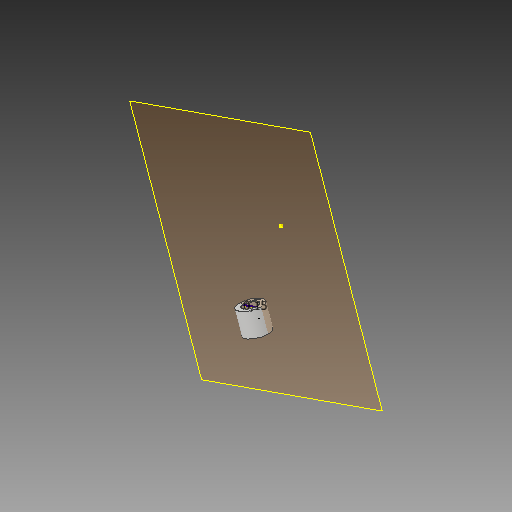
# Autodesk Inventor part: motor_handler
Saved by Autodesk Inventor 2019 (Build 230136000, 136)
## iProperties
Created: 2019-01-23
Part Number: motor_handler
Material: Generic
Document SubType Name: Modeling
Designer: jmc
Density: 1 g/cm^3
Appearance: Default
Author: jmc
Autodesk Inventor part; units mm, degrees
ref_plane "YZ Plane" through (0, 0, 0) normal (1, 0, 0) x (0, 1, 0)
ref_plane "XZ Plane" through (0, 0, 0) normal (0, 1, 0) x (-1, 0, 0)
ref_plane "XY Plane" through (0, 0, 0) normal (0, 0, 1) x (1, 0, 0)
ref_plane "Work Plane2" through (-89.4914, 16.4002, -46.0725) normal (0, 0, 1) x (0.3299211, -0.9440085, 0)
sketch "Sketch3" plane through (-89.4914, 16.4002, -46.0725) normal (0, 0, 1) x (0.3299211, -0.9440085, 0)
  line L0 (142.5, 12.3) -> (142.5, -12.3) projected
  line L1 (142.35, 11.9681) -> (142.35, -12.4873)
  point P0 (45.0071, 79.0699)
  dimension "d3" = 0.15
  constraints: 2 end point, 1 vertical
  measures "d3" distance between parallel lines of L1 L0
sketch "Sketch2" plane through (-89.4914, 16.4002, -46.0725) normal (0, 0, 1) x (0.3299211, -0.9440085, 0)
  line L0 (144.2, -14) -> (171.4, -14)
  line L1 (142.5, -12.3) -> (142.5, 11.0344) projected
  line L2 (130, 22) -> (130, -22) projected
  line L3 (144.2, 16.15) -> (171.4, 16.15)
  line L4 (171.4, 16.15) -> (171.4, 14.15)
  line L5 (144.2, 14.15) -> (171.4, 14.15)
  line L6 (156.1685, 0) -> (84.745, 0) construction
  line L7 (144.2, 14.15) -> (142.35, 14.15)
  line L8 (142.35, 16.15) -> (144.2, 16.15)
  line L9 (142.35, 11.9681) -> (142.35, -12.4873) projected
  line L10 (142.5, 14.15) -> (142.35, 14.15)
  line L11 (142.35, 14.15) -> (142.35, 16.15)
  line L12 (142.35, 16.15) -> (142.5, 16.15)
  point P0 (45.0071, 79.0699)
  dimension "d7" = 2
  constraints: 18 end point, 4 perpendicular, 3 horizontal, 2 point on line, 1 collinear, 4 other
  measures "d7" distance between parallel lines of L5 L3
revolve "Revolution1" add sketch "Sketch2" angle 360 about axis through (-37.9682, -131.0241, -46.0725) along (-0.3299211, 0.9440085, 0)
sketch "Sketch4" plane through (-42.5272, -117.9794, -46.0725) normal (-0.3299211, 0.9440085, 0) x (0.9440085, 0.3299211, 0)
  circle A0 centre (0, 0) radius 10
  circle A1 centre (0, 0) radius 16.15
  point P0 (79.0699, -46.0725)
  dimension "d4" = 20
  constraints: 2 centre point, 1 coincident
  measures "d4" diameter of A0
extrude "Extrusion2" add sketch "Sketch4" along normal blind 1
body "Solid1"
